Autodesk Fusion 360 part; units mm, degrees
note: some values were not read from the file. Chosen so that the rebuilt part matches the saved one: which bodies a step acts on; which face or edge a step refers to. Set by a fixed rule: which sketch regions a step uses.
(part 2 of 3)
sketch "Sketch13" plane through (0, 0, 15) normal (0, 0, 1) x (-1, 0, 0)
  line L0 (-263, -205.6688) -> (-253, -205.6688)
  line L1 (-253, -205.6688) -> (-253, -217.3312)
  line L2 (-253, -217.3312) -> (-263, -217.3312)
  line L3 (-263, -217.3312) -> (-263, -205.6688)
  line L4 (-263, -137.6688) -> (-253, -137.6688)
  line L5 (-253, -137.6688) -> (-253, -149.3312)
  line L6 (-253, -149.3312) -> (-263, -149.3312)
  line L7 (-263, -149.3312) -> (-263, -137.6688)
  line L8 (-263, -69.6688) -> (-253, -69.6688)
  line L9 (-253, -69.6688) -> (-253, -81.3312)
  line L10 (-253, -81.3312) -> (-263, -81.3312)
  line L11 (-263, -81.3312) -> (-263, -69.6688)
  line L12 (-263, -4) -> (-253, -4)
  line L13 (-253, -4) -> (-253, -13.3312)
  line L14 (-253, -13.3312) -> (-263, -13.3312)
  line L15 (-263, -13.3312) -> (-263, -4)
  line L16 (-263, -52.6688) -> (-253, -52.6688)
  line L17 (-253, -52.6688) -> (-253, -64.3312)
  line L18 (-253, -64.3312) -> (-263, -64.3312)
  line L19 (-263, -64.3312) -> (-263, -52.6688)
  line L20 (-263, -120.6688) -> (-253, -120.6688)
  line L21 (-253, -120.6688) -> (-253, -132.3312)
  line L22 (-253, -132.3312) -> (-263, -132.3312)
  line L23 (-263, -132.3312) -> (-263, -120.6688)
  line L24 (-263, -188.6688) -> (-253, -188.6688)
  line L25 (-253, -188.6688) -> (-253, -200.3312)
  line L26 (-253, -200.3312) -> (-263, -200.3312)
  line L27 (-263, -200.3312) -> (-263, -188.6688)
  line L28 (-263, -222.6688) -> (-253, -222.6688)
  line L29 (-253, -222.6688) -> (-253, -234.3312)
  line L30 (-253, -234.3312) -> (-263, -234.3312)
  line L31 (-263, -234.3312) -> (-263, -222.6688)
  line L32 (-263, -154.6688) -> (-253, -154.6688)
  line L33 (-253, -154.6688) -> (-253, -166.3312)
  line L34 (-253, -166.3312) -> (-263, -166.3312)
  line L35 (-263, -166.3312) -> (-263, -154.6688)
  line L36 (-263, -86.6688) -> (-253, -86.6688)
  line L37 (-253, -86.6688) -> (-253, -98.3312)
  line L38 (-253, -98.3312) -> (-263, -98.3312)
  line L39 (-263, -98.3312) -> (-263, -86.6688)
  line L40 (-263, -18.6688) -> (-253, -18.6688)
  line L41 (-253, -18.6688) -> (-253, -30.3312)
  line L42 (-253, -30.3312) -> (-263, -30.3312)
  line L43 (-263, -30.3312) -> (-263, -18.6688)
  line L44 (-263, -35.6688) -> (-253, -35.6688)
  line L45 (-253, -35.6688) -> (-253, -47.3312)
  line L46 (-253, -47.3312) -> (-263, -47.3312)
  line L47 (-263, -47.3312) -> (-263, -35.6688)
  line L48 (-263, -103.6688) -> (-253, -103.6688)
  line L49 (-253, -103.6688) -> (-253, -115.3312)
  line L50 (-253, -115.3312) -> (-263, -115.3312)
  line L51 (-263, -115.3312) -> (-263, -103.6688)
  line L52 (-263, -171.6688) -> (-253, -171.6688)
  line L53 (-253, -171.6688) -> (-253, -183.3312)
  line L54 (-253, -183.3312) -> (-263, -183.3312)
  line L55 (-263, -183.3312) -> (-263, -171.6688)
  line L56 (-263, -239.6688) -> (-253, -239.6688)
  line L57 (-253, -239.6688) -> (-253, -247)
  line L58 (-253, -247) -> (-263, -247)
  line L59 (-263, -247) -> (-263, -239.6688)
  line L60 (-297, -205.6688) -> (-287, -205.6688)
  line L61 (-287, -205.6688) -> (-287, -217.3312)
  line L62 (-287, -217.3312) -> (-297, -217.3312)
  line L63 (-297, -217.3312) -> (-297, -205.6688)
  line L64 (-297, -137.6688) -> (-287, -137.6688)
  line L65 (-287, -137.6688) -> (-287, -149.3312)
  line L66 (-287, -149.3312) -> (-297, -149.3312)
  line L67 (-297, -149.3312) -> (-297, -137.6688)
  line L68 (-297, -69.6688) -> (-287, -69.6688)
  line L69 (-287, -69.6688) -> (-287, -81.3312)
  line L70 (-287, -81.3312) -> (-297, -81.3312)
  line L71 (-297, -81.3312) -> (-297, -69.6688)
  line L72 (-297, -4) -> (-287, -4)
  line L73 (-287, -4) -> (-287, -13.3312)
  line L74 (-287, -13.3312) -> (-297, -13.3312)
  line L75 (-297, -13.3312) -> (-297, -4)
  line L76 (-297, -52.6688) -> (-287, -52.6688)
  line L77 (-287, -52.6688) -> (-287, -64.3312)
  line L78 (-287, -64.3312) -> (-297, -64.3312)
  line L79 (-297, -64.3312) -> (-297, -52.6688)
  line L80 (-297, -120.6688) -> (-287, -120.6688)
  line L81 (-287, -120.6688) -> (-287, -132.3312)
  line L82 (-287, -132.3312) -> (-297, -132.3312)
  line L83 (-297, -132.3312) -> (-297, -120.6688)
  line L84 (-297, -188.6688) -> (-287, -188.6688)
  line L85 (-287, -188.6688) -> (-287, -200.3312)
  line L86 (-287, -200.3312) -> (-297, -200.3312)
  line L87 (-297, -200.3312) -> (-297, -188.6688)
  line L88 (-297, -222.6688) -> (-287, -222.6688)
  line L89 (-287, -222.6688) -> (-287, -234.3312)
  line L90 (-287, -234.3312) -> (-297, -234.3312)
  line L91 (-297, -234.3312) -> (-297, -222.6688)
  line L92 (-297, -154.6688) -> (-287, -154.6688)
  line L93 (-287, -154.6688) -> (-287, -166.3312)
  line L94 (-287, -166.3312) -> (-297, -166.3312)
  line L95 (-297, -166.3312) -> (-297, -154.6688)
  line L96 (-297, -86.6688) -> (-287, -86.6688)
  line L97 (-287, -86.6688) -> (-287, -98.3312)
  line L98 (-287, -98.3312) -> (-297, -98.3312)
  line L99 (-297, -98.3312) -> (-297, -86.6688)
  line L100 (-297, -18.6688) -> (-287, -18.6688)
  line L101 (-287, -18.6688) -> (-287, -30.3312)
  line L102 (-287, -30.3312) -> (-297, -30.3312)
  line L103 (-297, -30.3312) -> (-297, -18.6688)
  line L104 (-297, -35.6688) -> (-287, -35.6688)
  line L105 (-287, -35.6688) -> (-287, -47.3312)
  line L106 (-287, -47.3312) -> (-297, -47.3312)
  line L107 (-297, -47.3312) -> (-297, -35.6688)
  line L108 (-297, -103.6688) -> (-287, -103.6688)
  line L109 (-287, -103.6688) -> (-287, -115.3312)
  line L110 (-287, -115.3312) -> (-297, -115.3312)
  line L111 (-297, -115.3312) -> (-297, -103.6688)
  line L112 (-297, -171.6688) -> (-287, -171.6688)
  line L113 (-287, -171.6688) -> (-287, -183.3312)
  line L114 (-287, -183.3312) -> (-297, -183.3312)
  line L115 (-297, -183.3312) -> (-297, -171.6688)
  line L116 (-297, -239.6688) -> (-287, -239.6688)
  line L117 (-287, -239.6688) -> (-287, -247)
  line L118 (-287, -247) -> (-297, -247)
  line L119 (-297, -247) -> (-297, -239.6688)
  line L120 (-250, -250) -> (-250, 0)
  line L121 (-250, 0) -> (-300, 0)
  line L122 (-300, 0) -> (-300, -250)
  line L123 (-300, -250) -> (-250, -250)
  line L124 (-257.25, -13.3312) -> (-258.75, -13.3312)
  line L125 (-258.75, -13.3312) -> (-258.75, -154.6688)
  line L126 (-257.25, -13.3312) -> (-257.25, -154.6688)
  line L127 (-258.75, -154.6688) -> (-257.25, -154.6688)
  line L128 (-292.75, -103.6688) -> (-292.75, -239.6688)
  line L129 (-291.25, -103.6688) -> (-291.25, -239.6688)
  line L130 (-292.75, -239.6688) -> (-291.25, -239.6688)
  line L131 (-291.25, -103.6688) -> (-291.25, -98.3312)
  line L132 (-292.75, -103.6688) -> (-292.75, -98.3312)
  line L133 (-292.75, -98.3312) -> (-291.25, -98.3312)
  dimension "d115" = 4.25
  dimension "d120" = 1.5
  dimension "d121" = 1.5
  dimension "d144" = 1.5
  constraint coincident L14 L124.start
  constraint coincident L14 L124.end
  constraint coincident L32 L125.end
  constraint perpendicular L32 L125
  constraint coincident L32 L126.end
  constraint coincident L108 L128.start
  constraint coincident L108 L129.start
  constraint coincident L116 L128.end
  constraint perpendicular L116 L128
  constraint coincident L116 L129.end
  constraint perpendicular L116 L129
  constraint coincident L98 L131.end
  constraint perpendicular L98 L131
  constraint coincident L98 L132.end
  constraint perpendicular L98 L132
  measures "d115" distance of L14.end L124.end
  measures "d120" distance of L125.end L126.end
  measures "d121" distance of L124.start L124.end
  measures "d144" distance of L131.end L132.end
extrude "Extrude15" cut sketch "Sketch13" against normal blind 1 contours L4 L22 L125 L126 | L4 L6 L125 L126 | L20 L22 L125 L126 | L6 L32 L125 L126 L127 | L20 L50 L125 L126 | L48 L50 L125 L126 | L38 L48 L125 L126 | L36 L38 L125 L126 | L10 L36 L125 L126 | L8 L10 L125 L126 | L8 L18 L125 L126 | L16 L18 L125 L126 | L16 L46 L125 L126 | L44 L46 L125 L126 | L42 L44 L125 L126 | L40 L42 L125 L126 | L14 L40 L124 L125 L126 | L60 L86 L128 L129 | L60 L62 L128 L129 | L84 L86 L128 L129 | L62 L88 L128 L129 | L84 L114 L128 L129 | L88 L90 L128 L129 | L112 L114 L128 L129 | L90 L116 L128 L129 L130 | L94 L112 L128 L129 | L92 L94 L128 L129 | L66 L92 L128 L129 | L64 L66 L128 L129 | L64 L82 L128 L129 | L80 L82 L128 L129 | L80 L110 L128 L129 | L108 L110 L128 L129 | L98 L108 L131 L132 L133 bodies 39
sketch "Sketch14" plane through (0, 0, 15) normal (0, 0, 1) x (-1, 0, 0)
  line L0 (-258.75, -154.6688) -> (-258.75, -149.3312)
  line L1 (-258.75, -149.3312) -> (-263, -149.3312)
  line L2 (-263, -149.3312) -> (-263, -137.6688)
  line L3 (-263, -137.6688) -> (-258.75, -137.6688)
  line L4 (-258.75, -137.6688) -> (-258.75, -132.3312)
  line L5 (-258.75, -132.3312) -> (-263, -132.3312)
  line L6 (-263, -132.3312) -> (-263, -120.6688)
  line L7 (-263, -120.6688) -> (-258.75, -120.6688)
  line L8 (-258.75, -120.6688) -> (-258.75, -115.3312)
  line L9 (-258.75, -115.3312) -> (-263, -115.3312)
  line L10 (-263, -115.3312) -> (-263, -103.6688)
  line L11 (-263, -103.6688) -> (-258.75, -103.6688)
  line L12 (-258.75, -103.6688) -> (-258.75, -98.3312)
  line L13 (-258.75, -98.3312) -> (-263, -98.3312)
  line L14 (-263, -98.3312) -> (-263, -86.6688)
  line L15 (-263, -86.6688) -> (-258.75, -86.6688)
  line L16 (-258.75, -86.6688) -> (-258.75, -81.3312)
  line L17 (-258.75, -81.3312) -> (-263, -81.3312)
  line L18 (-263, -81.3312) -> (-263, -69.6688)
  line L19 (-263, -69.6688) -> (-258.75, -69.6688)
  line L20 (-258.75, -69.6688) -> (-258.75, -64.3312)
  line L21 (-258.75, -64.3312) -> (-263, -64.3312)
  line L22 (-263, -64.3312) -> (-263, -52.6688)
  line L23 (-263, -52.6688) -> (-258.75, -52.6688)
  line L24 (-258.75, -52.6688) -> (-258.75, -47.3312)
  line L25 (-258.75, -47.3312) -> (-263, -47.3312)
  line L26 (-263, -47.3312) -> (-263, -35.6688)
  line L27 (-263, -35.6688) -> (-258.75, -35.6688)
  line L28 (-258.75, -35.6688) -> (-258.75, -30.3312)
  line L29 (-258.75, -30.3312) -> (-263, -30.3312)
  line L30 (-263, -30.3312) -> (-263, -18.6688)
  line L31 (-263, -18.6688) -> (-258.75, -18.6688)
  line L32 (-258.75, -18.6688) -> (-258.75, -13.3312)
  line L33 (-258.75, -13.3312) -> (-263, -13.3312)
  line L34 (-263, -13.3312) -> (-263, -4)
  line L35 (-263, -4) -> (-253, -4)
  line L36 (-253, -4) -> (-253, -13.3312)
  line L37 (-253, -13.3312) -> (-257.25, -13.3312)
  line L38 (-257.25, -13.3312) -> (-257.25, -18.6688)
  line L39 (-257.25, -18.6688) -> (-253, -18.6688)
  line L40 (-253, -18.6688) -> (-253, -30.3312)
  line L41 (-253, -30.3312) -> (-257.25, -30.3312)
  line L42 (-257.25, -30.3312) -> (-257.25, -35.6688)
  line L43 (-257.25, -35.6688) -> (-253, -35.6688)
  line L44 (-253, -35.6688) -> (-253, -47.3312)
  line L45 (-253, -47.3312) -> (-257.25, -47.3312)
  line L46 (-257.25, -47.3312) -> (-257.25, -52.6688)
  line L47 (-257.25, -52.6688) -> (-253, -52.6688)
  line L48 (-253, -52.6688) -> (-253, -64.3312)
  line L49 (-253, -64.3312) -> (-257.25, -64.3312)
  line L50 (-257.25, -64.3312) -> (-257.25, -69.6688)
  line L51 (-257.25, -69.6688) -> (-253, -69.6688)
  line L52 (-253, -69.6688) -> (-253, -81.3312)
  line L53 (-253, -81.3312) -> (-257.25, -81.3312)
  line L54 (-257.25, -81.3312) -> (-257.25, -86.6688)
  line L55 (-257.25, -86.6688) -> (-253, -86.6688)
  line L56 (-253, -86.6688) -> (-253, -98.3312)
  line L57 (-253, -98.3312) -> (-257.25, -98.3312)
  line L58 (-257.25, -98.3312) -> (-257.25, -103.6688)
  line L59 (-257.25, -103.6688) -> (-253, -103.6688)
  line L60 (-253, -103.6688) -> (-253, -115.3312)
  line L61 (-253, -115.3312) -> (-257.25, -115.3312)
  line L62 (-257.25, -115.3312) -> (-257.25, -120.6688)
  line L63 (-257.25, -120.6688) -> (-253, -120.6688)
  line L64 (-253, -120.6688) -> (-253, -132.3312)
  line L65 (-253, -132.3312) -> (-257.25, -132.3312)
  line L66 (-257.25, -132.3312) -> (-257.25, -137.6688)
  line L67 (-257.25, -137.6688) -> (-253, -137.6688)
  line L68 (-253, -137.6688) -> (-253, -149.3312)
  line L69 (-253, -149.3312) -> (-257.25, -149.3312)
  line L70 (-257.25, -149.3312) -> (-257.25, -154.6688)
  line L71 (-257.25, -154.6688) -> (-253, -154.6688)
  line L72 (-253, -154.6688) -> (-253, -166.3312)
  line L73 (-253, -166.3312) -> (-263, -166.3312)
  line L74 (-263, -166.3312) -> (-263, -154.6688)
  line L75 (-263, -154.6688) -> (-258.75, -154.6688)
  line L76 (-263, -205.6688) -> (-253, -205.6688)
  line L77 (-253, -205.6688) -> (-253, -217.3312)
  line L78 (-253, -217.3312) -> (-263, -217.3312)
  line L79 (-263, -217.3312) -> (-263, -205.6688)
  line L80 (-263, -188.6688) -> (-253, -188.6688)
  line L81 (-253, -188.6688) -> (-253, -200.3312)
  line L82 (-253, -200.3312) -> (-263, -200.3312)
  line L83 (-263, -200.3312) -> (-263, -188.6688)
  line L84 (-263, -222.6688) -> (-253, -222.6688)
  line L85 (-253, -222.6688) -> (-253, -234.3312)
  line L86 (-253, -234.3312) -> (-263, -234.3312)
  line L87 (-263, -234.3312) -> (-263, -222.6688)
  line L88 (-263, -171.6688) -> (-253, -171.6688)
  line L89 (-253, -171.6688) -> (-253, -183.3312)
  line L90 (-253, -183.3312) -> (-263, -183.3312)
  line L91 (-263, -183.3312) -> (-263, -171.6688)
  line L92 (-263, -239.6688) -> (-253, -239.6688)
  line L93 (-253, -239.6688) -> (-253, -247)
  line L94 (-253, -247) -> (-263, -247)
  line L95 (-263, -247) -> (-263, -239.6688)
  line L96 (-297, -69.6688) -> (-287, -69.6688)
  line L97 (-287, -69.6688) -> (-287, -81.3312)
  line L98 (-287, -81.3312) -> (-297, -81.3312)
  line L99 (-297, -81.3312) -> (-297, -69.6688)
  line L100 (-297, -4) -> (-287, -4)
  line L101 (-287, -4) -> (-287, -13.3312)
  line L102 (-287, -13.3312) -> (-297, -13.3312)
  line L103 (-297, -13.3312) -> (-297, -4)
  line L104 (-297, -52.6688) -> (-287, -52.6688)
  line L105 (-287, -52.6688) -> (-287, -64.3312)
  line L106 (-287, -64.3312) -> (-297, -64.3312)
  line L107 (-297, -64.3312) -> (-297, -52.6688)
  line L108 (-297, -86.6688) -> (-287, -86.6688)
  line L109 (-287, -86.6688) -> (-287, -98.3312)
  line L110 (-292.75, -98.3312) -> (-297, -98.3312)
  line L111 (-297, -98.3312) -> (-297, -86.6688)
  line L112 (-297, -18.6688) -> (-287, -18.6688)
  line L113 (-287, -18.6688) -> (-287, -30.3312)
  line L114 (-287, -30.3312) -> (-297, -30.3312)
  line L115 (-297, -30.3312) -> (-297, -18.6688)
  line L116 (-297, -35.6688) -> (-287, -35.6688)
  line L117 (-287, -35.6688) -> (-287, -47.3312)
  line L118 (-287, -47.3312) -> (-297, -47.3312)
  line L119 (-297, -47.3312) -> (-297, -35.6688)
  line L120 (-292.75, -137.6688) -> (-292.75, -132.3312)
  line L121 (-292.75, -132.3312) -> (-297, -132.3312)
  line L122 (-297, -132.3312) -> (-297, -120.6688)
  line L123 (-297, -120.6688) -> (-292.75, -120.6688)
  line L124 (-292.75, -120.6688) -> (-292.75, -115.3312)
  line L125 (-292.75, -115.3312) -> (-297, -115.3312)
  line L126 (-297, -115.3312) -> (-297, -103.6688)
  line L127 (-297, -103.6688) -> (-292.75, -103.6688)
  line L128 (-287, -103.6688) -> (-287, -115.3312)
  line L129 (-287, -115.3312) -> (-291.25, -115.3312)
  line L130 (-291.25, -98.3312) -> (-291.25, -103.6688)
  line L131 (-291.25, -120.6688) -> (-287, -120.6688)
  line L132 (-287, -120.6688) -> (-287, -132.3312)
  line L133 (-287, -132.3312) -> (-291.25, -132.3312)
  line L134 (-291.25, -132.3312) -> (-291.25, -137.6688)
  line L135 (-291.25, -137.6688) -> (-287, -137.6688)
  line L136 (-287, -137.6688) -> (-287, -149.3312)
  line L137 (-287, -149.3312) -> (-291.25, -149.3312)
  line L138 (-291.25, -149.3312) -> (-291.25, -154.6688)
  line L139 (-291.25, -154.6688) -> (-287, -154.6688)
  line L140 (-287, -154.6688) -> (-287, -166.3312)
  line L141 (-287, -166.3312) -> (-291.25, -166.3312)
  line L142 (-291.25, -166.3312) -> (-291.25, -171.6688)
  line L143 (-291.25, -171.6688) -> (-287, -171.6688)
  line L144 (-287, -171.6688) -> (-287, -183.3312)
  line L145 (-287, -183.3312) -> (-291.25, -183.3312)
  line L146 (-291.25, -183.3312) -> (-291.25, -188.6688)
  line L147 (-291.25, -188.6688) -> (-287, -188.6688)
  line L148 (-287, -188.6688) -> (-287, -200.3312)
  line L149 (-287, -200.3312) -> (-291.25, -200.3312)
  line L150 (-291.25, -200.3312) -> (-291.25, -205.6688)
  line L151 (-291.25, -205.6688) -> (-287, -205.6688)
  line L152 (-287, -205.6688) -> (-287, -217.3312)
  line L153 (-287, -217.3312) -> (-291.25, -217.3312)
  line L154 (-291.25, -217.3312) -> (-291.25, -222.6688)
  line L155 (-291.25, -222.6688) -> (-287, -222.6688)
  line L156 (-287, -222.6688) -> (-287, -234.3312)
  line L157 (-287, -234.3312) -> (-291.25, -234.3312)
  line L158 (-291.25, -234.3312) -> (-291.25, -239.6688)
  line L159 (-291.25, -239.6688) -> (-287, -239.6688)
  line L160 (-287, -239.6688) -> (-287, -247)
  line L161 (-287, -247) -> (-297, -247)
  line L162 (-297, -247) -> (-297, -239.6688)
  line L163 (-297, -239.6688) -> (-292.75, -239.6688)
  line L164 (-292.75, -239.6688) -> (-292.75, -234.3312)
  line L165 (-292.75, -234.3312) -> (-297, -234.3312)
  line L166 (-297, -234.3312) -> (-297, -222.6688)
  line L167 (-297, -222.6688) -> (-292.75, -222.6688)
  line L168 (-292.75, -222.6688) -> (-292.75, -217.3312)
  line L169 (-292.75, -217.3312) -> (-297, -217.3312)
  line L170 (-297, -217.3312) -> (-297, -205.6688)
  line L171 (-297, -205.6688) -> (-292.75, -205.6688)
  line L172 (-292.75, -205.6688) -> (-292.75, -200.3312)
  line L173 (-292.75, -200.3312) -> (-297, -200.3312)
  line L174 (-297, -200.3312) -> (-297, -188.6688)
  line L175 (-297, -188.6688) -> (-292.75, -188.6688)
  line L176 (-292.75, -188.6688) -> (-292.75, -183.3312)
  line L177 (-292.75, -183.3312) -> (-297, -183.3312)
  line L178 (-297, -183.3312) -> (-297, -171.6688)
  line L179 (-297, -171.6688) -> (-292.75, -171.6688)
  line L180 (-292.75, -171.6688) -> (-292.75, -166.3312)
  line L181 (-292.75, -166.3312) -> (-297, -166.3312)
  line L182 (-297, -166.3312) -> (-297, -154.6688)
  line L183 (-297, -154.6688) -> (-292.75, -154.6688)
  line L184 (-292.75, -154.6688) -> (-292.75, -149.3312)
  line L185 (-292.75, -149.3312) -> (-297, -149.3312)
  line L186 (-297, -149.3312) -> (-297, -137.6688)
  line L187 (-297, -137.6688) -> (-292.75, -137.6688)
  line L188 (-250, -250) -> (-250, 0)
  line L189 (-250, 0) -> (-300, 0)
  line L190 (-300, 0) -> (-300, -250)
  line L191 (-300, -250) -> (-250, -250)
  line L192 (-297, -4) -> (-253, -4)
  line L193 (-253, -4) -> (-253, -247)
  line L194 (-253, -247) -> (-297, -247)
  line L195 (-297, -247) -> (-297, -4)
  line L196 (-252, -248) -> (-298, -248)
  line L197 (-298, -248) -> (-298, -3)
  line L198 (-298, -3) -> (-252, -3)
  line L199 (-252, -3) -> (-252, -248)
  line L200 (-287, -4) -> (-287, -247)
  line L201 (-263, -247) -> (-263, -4)
  line L202 (-286, -4) -> (-286, -247)
  line L203 (-264, -247) -> (-264, -4)
  line L204 (-292.75, -103.6688) -> (-292.75, -98.3312)
  line L205 (-287, -98.3312) -> (-291.25, -98.3312)
  line L206 (-291.25, -103.6688) -> (-287, -103.6688)
  line L207 (-291.25, -115.3312) -> (-291.25, -120.6688)
  dimension "d126" = -1
  dimension "d127" = -1
  dimension "d128" = -1
  constraint horizontal L192
  constraint vertical L193
  constraint horizontal L194
  constraint vertical L195
  constraint coincident L93.end L94.start
  constraint coincident L100.start L103.end
  constraint coincident L100.end L101.start
  constraint coincident L160.end L161.start
  constraint coincident L94.end L95.start
  constraint coincident L34.end L35.start
extrude "Extrude16" add sketch "Sketch14" along normal blind 1 contours L2 L6 L10 L14 L18 L22 L26 L30 L34 L74 L79 L83 L87 L91 L95 L192 L194 L201 L203 | L97 L101 L105 L109 L113 L117 L128 L132 L136 L140 L144 L148 L152 L156 L160 L192 L194 L200 L202 | L196 L197 L198 L199 bodies 39
sketch "Sketch15" plane through (0, 0, 15) normal (0, 0, 1) x (-1, 0, 0)
  line L0 (-286, -247) -> (-264, -247)
  line L1 (-264, -247) -> (-264, -4)
  line L2 (-264, -4) -> (-286, -4)
  line L3 (-286, -4) -> (-286, -247)
  line L4 (-287, -234.33) -> (-287, -239.6688)
  line L5 (-287, -239.6688) -> (-291.25, -239.6688)
  line L6 (-291.25, -239.6688) -> (-291.25, -234.33)
  line L7 (-287, -234.33) -> (-291.25, -234.33)
  line L8 (-288, -235.33) -> (-290.25, -235.33)
  line L9 (-290.25, -238.6688) -> (-290.25, -235.33)
  line L10 (-288, -238.6688) -> (-290.25, -238.6688)
  line L11 (-288, -235.33) -> (-288, -238.6688)
  line L12 (-256.25, -153.6688) -> (-256.25, -150.33)
  line L13 (-254, -150.33) -> (-254, -153.6688)
  line L14 (-253, -149.33) -> (-253, -154.6688)
  line L15 (-253, -154.6688) -> (-257.25, -154.6688)
  line L16 (-254, -150.33) -> (-256.25, -150.33)
  line L17 (-253, -149.33) -> (-257.25, -149.33)
  line L18 (-257.25, -154.6688) -> (-257.25, -149.33)
  line L19 (-252, 81) -> (-252, -162)
  line L20 (-254, -153.6688) -> (-256.25, -153.6688)
  dimension "d131" = 5.3388
  dimension "d132" = 4.25
  dimension "d134" = 1
  dimension "d141" = 1
  dimension "d142" = 5.3388
  dimension "d143" = 4.25
  constraint parallel L3 L4
  constraint perpendicular L3 L5
  constraint perpendicular L5 L6
  constraint perpendicular L4 L7
  constraint parallel L14 L19
  constraint perpendicular L15 L19
  constraint perpendicular L15 L18
  constraint perpendicular L14 L17
  measures "d131" distance of L5.end L6.end
  measures "d132" distance of L4.start L6.end
  measures "d142" distance of L15.end L17.end
  measures "d143" distance of L14.start L17.end
extrude "Extrude17" add sketch "Sketch15" along normal blind 1 contours L8 L9 L10 L11 | L12 L13 L16 L20 bodies 39
pattern_linear "R-Pattern2" count 9 spacing 17 along (0, -1, 0) count 2 spacing 5.7 along (1, 0, 0) of "Extrude17"
sketch "Sketch16" plane through (0, 0, 0) normal (0, 0, -1) x (1, 0, 0)
  line L0 (300, -10) -> (300, 0)
  line L1 (300, 0) -> (287, 0)
  line L2 (300, 0) -> (250, 0)
  line L3 (250, 0) -> (250, -250)
  line L4 (250, -250) -> (300, -250)
  line L5 (300, -250) -> (300, 0)
  line L6 (246, 4) -> (246, -254)
  line L7 (246, -254) -> (304, -254)
  line L8 (304, -254) -> (304, 4)
  line L9 (304, 4) -> (246, 4)
  dimension "d145" = 4
  constraint horizontal L2
  constraint vertical L3
  constraint horizontal L4
  constraint vertical L5
  constraint coincident L0.end L1.start
extrude "Extrude18" add sketch "Sketch16" against normal blind 21 separate body contours L0 L1 L2 L3 L4 L5 | L6 L7 L8 L9 makes body 40
combine "Combine1'" operation cut target body 40 tool bodies 39 keep tools result as body 41 in component "Component"
move_body "Move4" bodies 39 to x (1, 0, 0) y (0, 1, 0) z (0, 0, 1) at (-22.6689, -7.9212, -52.6306)
split "Split3" by plane through (275, 125, 7.5) normal (1, 0, 0) bodies 40 makes body 42 at (284.6667, 82, 0)
move_body "Move1" bodies 41 to x (1, 0, 0) y (0, 1, 0) z (0, 0, 1) at (-137.3731, 35.75, -72.9165) in component "Component"
split "Split1" by plane through (112.6269, 35.75, -57.9165) normal (0, 0, -1) bodies 41 makes body 55 at (133.6269, 151.75, -72.9165) makes body 43 at (122.2936, 278.0879, -65.2499) makes body 54 at (118.9603, 267.412, -65.2499) makes body 53 at (118.9603, 244.0879, -65.2499) makes body 51 at (118.9603, 233.412, -65.2499) makes body 49 at (118.9603, 210.0879, -65.2499) makes body 47 at (118.9603, 199.412, -65.2499) makes body 47 at (120.3769, 114.2907, -65.5832) makes body 47 at (120.3769, 46.412, -65.2499) makes body 44 at (156.2936, 46.412, -65.2499) makes body 48 at (156.2936, 57.0879, -65.2499) makes body 46 at (156.2936, 74.0879, -65.2499) makes body 50 at (156.2936, 91.0879, -65.2499) makes body 52 at (156.2936, 114.412, -65.2499) makes body 45 at (156.2936, 125.0879, -65.2499) makes body 45 at (154.3769, 267.2907, -65.5832) makes body 45 at (154.8769, 278.0879, -65.2499) in component "Component"
move_body "Move2" bodies 55 to x (-1, 0, 0) y (0, 1, 0) z (0, 0, -1) at (190.1264, 20.1178, -160.1383) in component "Component"
delete_body "RemoveBody2" bodies 40
delete_body "RemoveBody3" bodies 42
ref_plane "WorkPlane4" through (52.4994, 180.8678, -47.2217) normal (0, 0, 1) x (-1, 0, 0)
combine "Combine2" operation add target body 47 tool bodies 41 45 44 48 43 49 52 46 51 53 50 54 in component "Component"
move_body "Move3" bodies 47 to x (1, 0, 0) y (0, -1, 0) z (0, 0, -1) at (0, 376.5599, -103.8331) in component "Component"
sketch "Sketch20" plane through (0, 0, -47.2217) normal (0, 0, 1) x (1, 0, 0)
  line L0 (77.4994, 55.8678) -> (27.4994, 55.8678)
  line L1 (27.4994, 55.8678) -> (27.4994, 305.8678)
  line L2 (27.4994, 305.8678) -> (77.4994, 305.8678)
  line L3 (77.4994, 305.8678) -> (77.4994, 55.8678)
  dimension "d153" = 50
  dimension "d154" = 250
  constraint horizontal L0
  constraint vertical L1
  constraint horizontal L2
  constraint vertical L3
  measures "d153" distance of L1.end L2.end
  measures "d154" distance of L0.end L1.end
extrude "Extrude20" add sketch "Sketch20" along normal blind 2.5 separate body makes body 56
fillet "Fillet1" radius 15 2 edges at (27.4994, 180.8678, -44.7217) (77.4994, 180.8678, -44.7217) on bodies 56
move_body "Move7" bodies 56 to x (-1, 0, 0) y (0, 1, 0) z (0, 0, -1) at (87.0021, 0, -89.4434)
sketch "Sketch22" plane through (0, 0, -42.2217) normal (0, 0, 1) x (-1, 0, 0)
  line L0 (-59.5027, -305.8678) -> (-9.5027, -305.8678)
  line L1 (-9.5027, -305.8678) -> (-9.5027, -55.8678)
  line L2 (-9.5027, -55.8678) -> (-59.5027, -55.8678)
  line L3 (-59.5027, -55.8678) -> (-59.5027, -305.8678)
  line L4 (-59.5027, -55.8678) -> (-9.5027, -55.8678)
  line L5 (-9.5027, -55.8678) -> (-9.5027, -305.8678)
  line L6 (-9.5027, -305.8678) -> (-59.5027, -305.8678)
  line L7 (-59.5027, -305.8678) -> (-59.5027, -55.8678)
  line L8 (-62.5027, -308.8678) -> (-62.5027, -52.8678)
  line L9 (-62.5027, -52.8678) -> (-6.5027, -52.8678)
  line L10 (-6.5027, -52.8678) -> (-6.5027, -308.8678)
  line L11 (-6.5027, -308.8678) -> (-62.5027, -308.8678)
  dimension "d160" = -3
  constraint horizontal L4
  constraint vertical L5
  constraint horizontal L6
  constraint vertical L7
  constraint coincident L0.end L1.start
  constraint coincident L2.end L3.start
extrude "Extrude22" add sketch "Sketch22" against normal blind 6 separate body contours L0 L1 L2 L3 L4 L5 L6 L7 | L8 L9 L10 L11 makes body 57
combine "Combine4" operation cut target body 57 tool bodies 56 keep tools
move_body "Move8" bodies 56 to x (-1, 0, 0) y (0, 1, 0) z (0, 0, -1) at (258.5331, -85.2699, -67.3692)
sketch "Sketch23" plane through (0, 0, -102.2217) normal (0, 0, -1) x (1, 0, 0)
  line L0 (77.4994, -305.8678) -> (27.4994, -305.8678)
  line L1 (27.4994, -305.8678) -> (27.4994, -55.8678)
  line L2 (27.4994, -55.8678) -> (77.4994, -55.8678)
  line L3 (77.4994, -55.8678) -> (77.4994, -305.8678)
  line L4 (81.4994, -309.8678) -> (81.4994, -51.8678)
  line L5 (81.4994, -51.8678) -> (23.4994, -51.8678)
  line L6 (23.4994, -51.8678) -> (23.4994, -309.8678)
  line L7 (23.4994, -309.8678) -> (81.4994, -309.8678)
  circle A0 centre (78.9994, -54.3678) radius 1
  circle A1 centre (25.9994, -54.3678) radius 1
  circle A2 centre (78.9994, -307.3678) radius 1
  circle A3 centre (25.9994, -307.3678) radius 1
  dimension "d163" = 2.5
  dimension "d164" = 2.5
  dimension "d165" = 2
  dimension "d168" = -53
  dimension "d169" = -253
  measures "d163" distance of L4 A0.centre
  measures "d164" distance of L5 A0.centre
  measures "d165" diameter of A0
extrude "Extrude1'" cut sketch "Sketch23" against normal blind 10 contours A0 | A1 | A2 | A3 bodies 55 in component "Component"
sketch "Sketch24" plane through (0, 0, -45.9166) normal (0, 0, 1) x (-1, 0, 0)
  line L0 (-108.6269, -344.81) -> (-108.6269, -86.81)
  line L1 (-108.6269, -86.81) -> (-166.6269, -86.81)
  line L2 (-166.6269, -86.81) -> (-166.6269, -344.81)
  line L3 (-166.6269, -344.81) -> (-108.6269, -344.81)
  line L4 (-114.6269, -92.81) -> (-114.6269, -337.81)
  line L5 (-114.6269, -337.81) -> (-160.6269, -337.81)
  line L6 (-160.6269, -337.81) -> (-160.6269, -92.81)
  line L7 (-160.6269, -92.81) -> (-114.6269, -92.81)
  circle A0 centre (-164.1269, -89.31) radius 0.925
  circle A1 centre (-111.1269, -89.31) radius 0.925
  circle A2 centre (-164.1269, -342.31) radius 0.925
  circle A3 centre (-111.1269, -342.31) radius 0.925
  dimension "d172" = 1.85
  dimension "d173" = 2.5
  dimension "d174" = 2.5
  dimension "d177" = 53
  dimension "d178" = -253
  measures "d172" diameter of A0
  measures "d173" distance of L1 A0.centre
  measures "d174" distance of L2 A0.centre
extrude "Extrude2'" add sketch "Sketch24" along normal blind 9.5 contours A0 | A1 | A2 | A3 bodies 47 in component "Component"
delete_body "RemoveBody4" bodies 38
delete_body "RemoveBody5" bodies 37
delete_body "RemoveBody6" bodies 36
delete_body "RemoveBody7" bodies 35
delete_body "RemoveBody8" bodies 34
delete_body "RemoveBody9" bodies 33
delete_body "RemoveBody10" bodies 32
delete_body "RemoveBody11" bodies 31
delete_body "RemoveBody12" bodies 30
delete_body "RemoveBody13" bodies 29
delete_body "RemoveBody14" bodies 28
delete_body "RemoveBody15" bodies 27
delete_body "RemoveBody16" bodies 26
delete_body "RemoveBody17" bodies 25
delete_body "RemoveBody18" bodies 24
delete_body "RemoveBody19" bodies 23
delete_body "RemoveBody20" bodies 22
delete_body "RemoveBody21" bodies 21
delete_body "RemoveBody22" bodies 20
delete_body "RemoveBody23" bodies 19
delete_body "RemoveBody24" bodies 18
delete_body "RemoveBody25" bodies 16
delete_body "RemoveBody26" bodies 17
delete_body "RemoveBody27" bodies 1
delete_body "RemoveBody28" bodies 11
delete_body "RemoveBody29" bodies 12
delete_body "RemoveBody30" bodies 13
delete_body "RemoveBody31" bodies 14
delete_body "RemoveBody32" bodies 15
move_body "Move4'" bodies 55 to x (1, 0, 0) y (0, 1, 0) z (0, 0, 1) at (85.0461, 34.5621, 56.9045) in component "Component"
move_body "Move10" bodies 56 to x (1, 0, 0) y (0, 1, 0) z (0, 0, 1) at (28.3007, 21.481, -12.4831)
move_body "Move6" bodies 55 to x (1, 0, 0) y (0, 1, 0) z (0, 0, 1) at (-25.3306, -90.1769, 49.3355) in component "Component"
move_body "Move11" bodies 56 to x (1, 0, 0) y (0, 1, 0) z (0, 0, 1) at (-235.3202, -99.4985, 135.8217)
move_body "Move12" bodies 56 to x (1, 0, 0) y (0, 1, 0) z (0, 0, 1) at (235, 100, -136)
move_body "Move13" bodies 56 to x (1, 0, 0) y (0, 1, 0) z (0, 0, 1) at (-212.7381, 45.3282, 54.3271)
extrude "Extrude23" add 5 faces at (236.9978, 160.1892, -37.6306) (233.6644, 177.1892, -37.6306) (233.6644, 194.1892, -37.6306) (233.6644, 211.1892, -37.6306) (233.6644, 228.1892, -37.6306) along direction (0, 0, 1) up to surface end surface through (-22.6689, -7.9212, -36.6306) normal (0, 0, 1) offset 0 on bodies 39 bodies 39
extrude "Extrude24" add 5 faces at (270.9978, 75.1892, -37.6306) (267.6644, 58.1892, -37.6306) (267.6644, 41.1892, -37.6306) (267.6644, 24.1892, -37.6306) (267.6644, 7.1892, -37.6306) along direction (0, 0, 1) up to surface end surface through (-22.6689, -7.9212, -36.6306) normal (0, 0, 1) offset 0 on bodies 39 bodies 39
extrude "Extrude25" add 1 faces at (248.6644, 77.0788, -37.6306) along direction (0, 0, 1) up to surface (1 mm away) on bodies 39 bodies 39
sketch "Sketch27" plane through (0, 0, -37.6306) normal (0, 0, 1) x (-1, 0, 0)
  line L0 (-227.3311, -242.0788) -> (-227.3311, 7.9212)
  line L1 (-227.3311, 7.9212) -> (-277.3311, 7.9212)
  line L2 (-277.3311, 7.9212) -> (-277.3311, -242.0788)
  line L3 (-277.3311, -242.0788) -> (-227.3311, -242.0788)
  line L4 (-229.3311, 4.9212) -> (-229.3311, -240.0788)
  line L5 (-229.3311, -240.0788) -> (-275.3311, -240.0788)
  line L6 (-275.3311, -240.0788) -> (-275.3311, 4.9212)
  line L7 (-275.3311, 4.9212) -> (-229.3311, 4.9212)
  line L8 (-285.3311, -250.0788) -> (-219.3311, -250.0788)
  line L9 (-219.3311, -250.0788) -> (-219.3311, 15.9212)
  line L10 (-219.3311, 15.9212) -> (-285.3311, 15.9212)
  line L11 (-285.3311, 15.9212) -> (-285.3311, -250.0788)
  dimension "d188" = 8
extrude "Extrude26" add sketch "Sketch27" against normal blind 2 contours L8 L9 L10 L11 bodies 39
sketch "Sketch28" plane through (0, 0, -37.6306) normal (0, 0, 1) x (-1, 0, 0)
  spline S0 degree 5 poles (-281, -14) (-281.6977, -14.6977) (-282.9408, -16.1019) (-284.349, -18.2348) (-285.3213, -21.0853) (-285.1001, -24.4243) (-283.6578, -27.3328) (-281.3643, -29.7132) (-279.0087, -31.8262) (-277.5287, -34.1742) (-277.2439, -36.9195) (-278.0887, -39.5081) (-279.3163, -41.6693) (-280.3953, -43.207) (-281, -44) knots 0 0 0 0 0 0 0.1 0.2 0.3 0.4 0.5 0.6 0.7 0.8 0.9 1 1 1 1 1 1
  spline S1 degree 5 poles (-281, -44) (-281.6977, -44.6977) (-282.9408, -46.1019) (-284.349, -48.2348) (-285.3213, -51.0853) (-285.1001, -54.4243) (-283.6578, -57.3328) (-281.3643, -59.7132) (-279.0087, -61.8262) (-277.5287, -64.1742) (-277.2439, -66.9195) (-278.0887, -69.5081) (-279.3163, -71.6693) (-280.3953, -73.207) (-281, -74) knots 0 0 0 0 0 0 0.1 0.2 0.3 0.4 0.5 0.6 0.7 0.8 0.9 1 1 1 1 1 1
  spline S2 degree 5 poles (-281, -74) (-281.6977, -74.6977) (-282.9408, -76.1019) (-284.349, -78.2348) (-285.3213, -81.0853) (-285.1001, -84.4243) (-283.6578, -87.3328) (-281.3643, -89.7132) (-279.0087, -91.8262) (-277.5287, -94.1742) (-277.2439, -96.9195) (-278.0887, -99.5081) (-279.3163, -101.6693) (-280.3953, -103.207) (-281, -104) knots 0 0 0 0 0 0 0.1 0.2 0.3 0.4 0.5 0.6 0.7 0.8 0.9 1 1 1 1 1 1
  spline S3 degree 5 poles (-281, -104) (-281.6977, -104.6977) (-282.9408, -106.1019) (-284.349, -108.2348) (-285.3213, -111.0853) (-285.1001, -114.4243) (-283.6578, -117.3328) (-281.3643, -119.7132) (-279.0087, -121.8262) (-277.5287, -124.1742) (-277.2439, -126.9195) (-278.0887, -129.5081) (-279.3163, -131.6693) (-280.3953, -133.207) (-281, -134) knots 0 0 0 0 0 0 0.1 0.2 0.3 0.4 0.5 0.6 0.7 0.8 0.9 1 1 1 1 1 1
  spline S4 degree 5 poles (-281, -134) (-281.6977, -134.6977) (-282.9408, -136.1019) (-284.349, -138.2348) (-285.3213, -141.0853) (-285.1001, -144.4243) (-283.6578, -147.3328) (-281.3643, -149.7132) (-279.0087, -151.8262) (-277.5287, -154.1742) (-277.2439, -156.9195) (-278.0887, -159.5081) (-279.3163, -161.6693) (-280.3953, -163.207) (-281, -164) knots 0 0 0 0 0 0 0.1 0.2 0.3 0.4 0.5 0.6 0.7 0.8 0.9 1 1 1 1 1 1
  spline S5 degree 5 poles (-281, -164) (-281.6977, -164.6977) (-282.9408, -166.1019) (-284.349, -168.2348) (-285.3213, -171.0853) (-285.1001, -174.4243) (-283.6578, -177.3328) (-281.3643, -179.7132) (-279.0087, -181.8262) (-277.5287, -184.1742) (-277.2439, -186.9195) (-278.0887, -189.5081) (-279.3163, -191.6693) (-280.3953, -193.207) (-281, -194) knots 0 0 0 0 0 0 0.1 0.2 0.3 0.4 0.5 0.6 0.7 0.8 0.9 1 1 1 1 1 1
  spline S6 degree 5 poles (-281, -194) (-281.6977, -194.6977) (-282.9408, -196.1019) (-284.349, -198.2348) (-285.3213, -201.0853) (-285.1001, -204.4243) (-283.6578, -207.3328) (-281.3643, -209.7132) (-279.0087, -211.8262) (-277.5287, -214.1742) (-277.2439, -216.9195) (-278.0887, -219.5081) (-279.3163, -221.6693) (-280.3953, -223.207) (-281, -224) knots 0 0 0 0 0 0 0.1 0.2 0.3 0.4 0.5 0.6 0.7 0.8 0.9 1 1 1 1 1 1
  spline S7 degree 5 poles (-281, -224) (-281.6977, -224.6977) (-282.9408, -226.1019) (-284.349, -228.2348) (-285.3213, -231.0853) (-285.1001, -234.4243) (-283.6578, -237.3328) (-281.3643, -239.7132) (-279.0087, -241.8262) (-277.5287, -244.1742) (-277.2439, -246.9195) (-278.0887, -249.5081) (-279.3163, -251.6693) (-280.3953, -253.207) (-281, -254) knots 0 0 0 0 0 0 0.1 0.2 0.3 0.4 0.5 0.6 0.7 0.8 0.9 1 1 1 1 1 1
  spline S8 degree 5 poles (-284.423, 11) (-283.9675, 11.6269) (-282.9967, 12.6902) (-281.3618, 13.7141) (-278.9468, 14.0495) (-276.163, 13.3548) (-274.1093, 12.1711) (-273.0331, 11.0447) (-272.0217, 9.9347) (-270.0405, 8.7409) (-267.3285, 8.0162) (-264.9659, 8.3194) (-263.3757, 9.3238) (-262.438, 10.3772) (-262, 11) knots 0 0 0 0 0 0 0.1 0.2 0.3 0.4 0.5 0.6 0.7 0.8 0.9 1 1 1 1 1 1
  line L0 (-274, 11.9999) -> (-272, 10.0001)
  spline S9 degree 5 poles (-284.423, 11) (-284.5806, 10.5896) (-284.9405, 9.4788) (-285.2295, 7.6931) (-284.9797, 5.3329) (-283.6578, 2.6672) (-281.3643, 0.2868) (-279.0087, -1.8262) (-277.5287, -4.1742) (-277.2439, -6.9195) (-278.0887, -9.5081) (-279.3163, -11.6693) (-280.3953, -13.207) (-281, -14) knots 0.141747 0.141747 0.141747 0.141747 0.141747 0.141747 0.2 0.3 0.4 0.5 0.6 0.7 0.8 0.9 1 1 1 1 1 1
  line L1 (-283.2517, 14.0516) -> (-285.5943, 7.9484)
  line L2 (-283.0208, 2.0208) -> (-278.9792, -2.0208)
  line L3 (-252.5, -250) -> (-252.5, -221)
  spline S10 degree 5 poles (-224, -14) (-223.3024, -14.6977) (-222.0592, -16.1019) (-220.651, -18.2348) (-219.6787, -21.0853) (-219.8999, -24.4243) (-221.3422, -27.3328) (-223.6357, -29.7132) (-225.9913, -31.8262) (-227.4713, -34.1742) (-227.7561, -36.9195) (-226.9113, -39.5081) (-225.6837, -41.6693) (-224.6047, -43.207) (-224, -44) knots 0 0 0 0 0 0 0.1 0.2 0.3 0.4 0.5 0.6 0.7 0.8 0.9 1 1 1 1 1 1
  line L4 (-277.7515, -10.7515) -> (-284.2485, -17.2485)
  line L5 (-277.8555, -39.8759) -> (-284.1445, -48.1241)
  line L6 (-227.2485, -10.7515) -> (-220.7515, -17.2485)
  line L7 (-227.1445, -39.8759) -> (-220.8555, -48.1241)
  spline S11 degree 5 poles (-224, -194) (-223.3024, -194.6977) (-222.0592, -196.1019) (-220.651, -198.2348) (-219.6787, -201.0853) (-219.8999, -204.4243) (-221.3422, -207.3328) (-223.6357, -209.7132) (-225.9913, -211.8262) (-227.4713, -214.1742) (-227.7561, -216.9195) (-226.9113, -219.5081) (-225.6837, -221.6693) (-224.6047, -223.207) (-224, -224) knots 0 0 0 0 0 0 0.1 0.2 0.3 0.4 0.5 0.6 0.7 0.8 0.9 1 1 1 1 1 1
  line L8 (-277.7515, -190.7515) -> (-284.2485, -197.2485)
  line L9 (-277.8555, -219.8759) -> (-284.1445, -228.1241)
  line L10 (-227.2485, -190.7515) -> (-220.7515, -197.2485)
  line L11 (-227.1445, -219.8759) -> (-220.8555, -228.1241)
  spline S12 degree 5 poles (-224, -104) (-223.3024, -104.6977) (-222.0592, -106.1019) (-220.651, -108.2348) (-219.6787, -111.0853) (-219.8999, -114.4243) (-221.3422, -117.3328) (-223.6357, -119.7132) (-225.9913, -121.8262) (-227.4713, -124.1742) (-227.7561, -126.9195) (-226.9113, -129.5081) (-225.6837, -131.6693) (-224.6047, -133.207) (-224, -134) knots 0 0 0 0 0 0 0.1 0.2 0.3 0.4 0.5 0.6 0.7 0.8 0.9 1 1 1 1 1 1
  line L12 (-277.7515, -100.7515) -> (-284.2485, -107.2485)
  line L13 (-277.8555, -129.8759) -> (-284.1445, -138.1241)
  line L14 (-227.2485, -100.7515) -> (-220.7515, -107.2485)
  line L15 (-227.1445, -129.8759) -> (-220.8555, -138.1241)
  spline S13 degree 5 poles (-224, -164) (-223.3024, -164.6977) (-222.0592, -166.1019) (-220.651, -168.2348) (-219.6787, -171.0853) (-219.8999, -174.4243) (-221.3422, -177.3328) (-223.6357, -179.7132) (-225.9913, -181.8262) (-227.4713, -184.1742) (-227.7561, -186.9195) (-226.9113, -189.5081) (-225.6837, -191.6693) (-224.6047, -193.207) (-224, -194) knots 0 0 0 0 0 0 0.1 0.2 0.3 0.4 0.5 0.6 0.7 0.8 0.9 1 1 1 1 1 1
  line L16 (-277.7515, -160.7515) -> (-284.2485, -167.2485)
  line L17 (-277.8555, -189.8759) -> (-284.1445, -198.1241)
  line L18 (-227.2485, -160.7515) -> (-220.7515, -167.2485)
  line L19 (-227.1445, -189.8759) -> (-220.8555, -198.1241)
  spline S14 degree 5 poles (-220.577, 11) (-220.4195, 10.5896) (-220.0595, 9.4788) (-219.7705, 7.6931) (-220.0203, 5.3329) (-221.3422, 2.6672) (-223.6357, 0.2868) (-225.9913, -1.8262) (-227.4713, -4.1742) (-227.7561, -6.9195) (-226.9113, -9.5081) (-225.6837, -11.6693) (-224.6047, -13.207) (-224, -14) knots 0.141747 0.141747 0.141747 0.141747 0.141747 0.141747 0.2 0.3 0.4 0.5 0.6 0.7 0.8 0.9 1 1 1 1 1 1
  line L20 (-278.1939, -10.3197) -> (-283.8061, -17.6803)
  line L21 (-221.7483, 14.0516) -> (-219.4057, 7.9484)
  line L22 (-221.9792, 2.0208) -> (-226.0208, -2.0208)
  line L23 (-226.8061, -10.3197) -> (-221.1939, -17.6803)
  spline S15 degree 5 poles (-224, -224) (-223.3024, -224.6977) (-222.0592, -226.1019) (-220.651, -228.2348) (-219.6787, -231.0853) (-219.8999, -234.4243) (-221.3422, -237.3328) (-223.6357, -239.7132) (-225.9913, -241.8262) (-227.4713, -244.1742) (-227.7561, -246.9195) (-226.9113, -249.5081) (-225.6837, -251.6693) (-224.6047, -253.207) (-224, -254) knots 0 0 0 0 0 0 0.1 0.2 0.3 0.4 0.5 0.6 0.7 0.8 0.9 1 1 1 1 1 1
  line L24 (-277.7515, -220.7515) -> (-284.2485, -227.2485)
  line L25 (-277.8555, -249.8759) -> (-284.1445, -258.1241)
  line L26 (-227.2485, -220.7515) -> (-220.7515, -227.2485)
  line L27 (-227.1445, -249.8759) -> (-220.8555, -258.1241)
  spline S16 degree 5 poles (-224, -44) (-223.3024, -44.6977) (-222.0592, -46.1019) (-220.651, -48.2348) (-219.6787, -51.0853) (-219.8999, -54.4243) (-221.3422, -57.3328) (-223.6357, -59.7132) (-225.9913, -61.8262) (-227.4713, -64.1742) (-227.7561, -66.9195) (-226.9113, -69.5081) (-225.6837, -71.6693) (-224.6047, -73.207) (-224, -74) knots 0 0 0 0 0 0 0.1 0.2 0.3 0.4 0.5 0.6 0.7 0.8 0.9 1 1 1 1 1 1
  line L28 (-277.7515, -40.7515) -> (-284.2485, -47.2485)
  line L29 (-277.8555, -69.8759) -> (-284.1445, -78.1241)
  line L30 (-227.2485, -40.7515) -> (-220.7515, -47.2485)
  line L31 (-227.1445, -69.8759) -> (-220.8555, -78.1241)
  spline S17 degree 5 poles (-224, -134) (-223.3024, -134.6977) (-222.0592, -136.1019) (-220.651, -138.2348) (-219.6787, -141.0853) (-219.8999, -144.4243) (-221.3422, -147.3328) (-223.6357, -149.7132) (-225.9913, -151.8262) (-227.4713, -154.1742) (-227.7561, -156.9195) (-226.9113, -159.5081) (-225.6837, -161.6693) (-224.6047, -163.207) (-224, -164) knots 0 0 0 0 0 0 0.1 0.2 0.3 0.4 0.5 0.6 0.7 0.8 0.9 1 1 1 1 1 1
  line L32 (-277.7515, -130.7515) -> (-284.2485, -137.2485)
  line L33 (-277.8555, -159.8759) -> (-284.1445, -168.1241)
  line L34 (-227.2485, -130.7515) -> (-220.7515, -137.2485)
  line L35 (-227.1445, -159.8759) -> (-220.8555, -168.1241)
  spline S18 degree 5 poles (-224, -74) (-223.3024, -74.6977) (-222.0592, -76.1019) (-220.651, -78.2348) (-219.6787, -81.0853) (-219.8999, -84.4243) (-221.3422, -87.3328) (-223.6357, -89.7132) (-225.9913, -91.8262) (-227.4713, -94.1742) (-227.7561, -96.9195) (-226.9113, -99.5081) (-225.6837, -101.6693) (-224.6047, -103.207) (-224, -104) knots 0 0 0 0 0 0 0.1 0.2 0.3 0.4 0.5 0.6 0.7 0.8 0.9 1 1 1 1 1 1
  line L36 (-277.7515, -70.7515) -> (-284.2485, -77.2485)
  line L37 (-277.8555, -99.8759) -> (-284.1445, -108.1241)
  line L38 (-227.2485, -70.7515) -> (-220.7515, -77.2485)
  line L39 (-227.1445, -99.8759) -> (-220.8555, -108.1241)
  spline S19 degree 5 poles (-220.577, 11) (-221.0325, 11.6269) (-222.0033, 12.6902) (-223.6382, 13.7141) (-226.0532, 14.0495) (-228.837, 13.3548) (-230.8907, 12.1711) (-231.9669, 11.0447) (-232.9783, 9.9347) (-234.9596, 8.7409) (-237.6716, 8.0162) (-240.0341, 8.3194) (-241.6243, 9.3238) (-242.562, 10.3772) (-243, 11) knots 0 0 0 0 0 0 0.1 0.2 0.3 0.4 0.5 0.6 0.7 0.8 0.9 1 1 1 1 1 1
  line L40 (-286.3297, 8.3759) -> (-282.5163, 13.6241)
  line L41 (-263.862, 8.3527) -> (-260.138, 13.6473)
  line L42 (-218.6703, 8.3759) -> (-222.4837, 13.6241)
  line L43 (-231, 11.9999) -> (-233, 10.0001)
  line L44 (-241.138, 8.3527) -> (-244.862, 13.6473)
  spline S20 degree 5 poles (-262, 11) (-261.6445, 11.3757) (-260.9314, 12.094) (-259.8553, 13.0722) (-258.4073, 14.1745) (-256.5738, 15.1934) (-254.7148, 15.8222) (-252.8284, 16.0305) (-250.9137, 15.8048) (-248.9719, 15.1654) (-247.0053, 14.145) (-245.4138, 13.0495) (-244.2106, 12.081) (-243.4042, 11.371) (-243, 11) knots 0 0 0 0 0 0 0.1 0.2 0.3 0.4 0.5 0.6 0.7 0.8 0.9 1 1 1 1 1 1
  line L45 (-219.3311, 15.9212) -> (-285.3311, 15.9212)
  line L46 (-281, -254) -> (-224, -254)
  line L47 (-295, 25) -> (-210, 25)
  line L48 (-210, 25) -> (-210, -260)
  line L49 (-210, -260) -> (-295, -260)
  line L50 (-295, -260) -> (-295, 25)
  point P0 (-281, 0)
  point P1 (-279, -32)
  point P2 (-281, -30)
  point P3 (-279, -62)
  point P4 (-281, -60)
  point P5 (-279, -92)
  point P6 (-281, -90)
  point P7 (-279, -122)
  point P8 (-281, -120)
  point P9 (-279, -152)
  point P10 (-281, -150)
  point P11 (-279, -182)
  point P12 (-281, -180)
  point P13 (-279, -212)
  point P14 (-281, -210)
  point P15 (-279, -242)
  point P16 (-281, -240)
  point P17 (-273, 11)
  point P18 (-226, -182)
  point P19 (-220, -250)
  point P20 (-232, 11)
  point P21 (-224, -180)
  point P22 (-226, -32)
  point P23 (-226, -122)
  point P24 (-224, -150)
  point P25 (-224, -90)
  point P26 (-224, 0)
  point P27 (-224, -120)
  point P28 (-224, -60)
  point P29 (-226, -152)
  point P30 (-226, -92)
  point P31 (-226, -242)
  point P32 (-226, -212)
  point P33 (-224, -210)
  point P34 (-224, 16)
  point P35 (-226, -62)
  point P36 (-224, -240)
  point P37 (-224, -30)
  point P38 (-253, 15.9212)
  dimension "d202" = 57
  constraint midpoint P17 L0
  constraint midpoint S8.start L1
  constraint midpoint P0 L2
  constraint midpoint S0.start L4
  constraint midpoint S0.end L5
  constraint midpoint S5.end L8
  constraint midpoint S6.end L9
  constraint midpoint S2.end L12
  constraint midpoint S3.end L13
  constraint midpoint S4.end L16
  constraint midpoint S5.end L17
  constraint midpoint S0.start L20
  constraint midpoint S6.end L24
  constraint midpoint S7.end L25
  constraint midpoint S0.end L28
  constraint midpoint S1.end L29
  constraint midpoint S3.end L32
  constraint midpoint S4.end L33
  constraint midpoint S1.end L36
  constraint midpoint S2.end L37
  constraint midpoint S8.start L40
  constraint midpoint S8.end L41
  constraint symmetric S0.start L3 S10.start
  constraint symmetric P0 L3 P26
  constraint symmetric P1 L3 P22
  constraint symmetric P2 L3 P37
  constraint symmetric S0.end L3 S10.end
  constraint symmetric P3 L3 P35
  constraint symmetric P4 L3 P28
  constraint symmetric S1.end L3 S16.end
  constraint symmetric P5 L3 P30
  constraint symmetric P6 L3 P25
  constraint symmetric S2.end L3 S12.start
  constraint symmetric P7 L3 P23
  constraint symmetric P8 L3 P27
  constraint symmetric S3.end L3 S12.end
  constraint symmetric P9 L3 P29
  constraint symmetric P10 L3 P24
  constraint symmetric S4.end L3 S13.start
  constraint symmetric P11 L3 P18
  constraint symmetric P12 L3 P21
  constraint symmetric S5.end L3 S11.start
  constraint symmetric P13 L3 P32
  constraint symmetric P14 L3 P33
  constraint symmetric S6.end L3 S11.end
  constraint symmetric P15 L3 P31
  constraint symmetric P16 L3 P36
  constraint symmetric S7.end L3 S15.end
  constraint symmetric S8.start L3 S14.start
  constraint symmetric S8.end L3 S19.end
  constraint symmetric P17 L3 P20
  constraint symmetric L0.start L3 L43.start
  constraint symmetric L0.end L3 L43.end
  constraint symmetric L1.start L3 L21.start
  constraint symmetric L1.end L3 L21.end
  constraint symmetric L2.start L3 L22.start
  constraint symmetric L2.end L3 L22.end
  constraint symmetric L3 L4.start L6.start
  constraint symmetric L3 L4.end L6.end
  constraint symmetric L3 L5.start L7.start
  constraint symmetric L3 L5.end L7.end
  constraint symmetric L3 L8.start L10.start
  constraint symmetric L3 L8.end L10.end
  constraint symmetric L3 L9.start L11.start
  constraint symmetric L3 L9.end L11.end
  constraint symmetric L3 L12.start L14.start
  constraint symmetric L3 L12.end L14.end
  constraint symmetric L3 L13.start L15.start
  constraint symmetric L3 L13.end L15.end
  constraint symmetric L3 L16.start L18.start
  constraint symmetric L3 L16.end L18.end
  constraint symmetric L3 L17.start L19.start
  constraint symmetric L3 L17.end L19.end
  constraint symmetric L3 L20.start L23.start
  constraint symmetric L3 L20.end L23.end
  constraint symmetric L3 L24.start L26.start
  constraint symmetric L3 L24.end L26.end
  constraint symmetric L3 L25.start L27.start
  constraint symmetric L3 L25.end L27.end
  constraint symmetric L3 L28.start L30.start
  constraint symmetric L3 L28.end L30.end
  constraint symmetric L3 L29.start L31.start
  constraint symmetric L3 L29.end L31.end
  constraint symmetric L3 L32.start L34.start
  constraint symmetric L3 L32.end L34.end
  constraint symmetric L3 L33.start L35.start
  constraint symmetric L3 L33.end L35.end
  constraint symmetric L3 L36.start L38.start
  constraint symmetric L3 L36.end L38.end
  constraint symmetric L3 L37.start L39.start
  constraint symmetric L3 L37.end L39.end
  constraint symmetric L3 L40.start L42.start
  constraint symmetric L3 L40.end L42.end
  constraint symmetric L3 L41.start L44.start
  constraint symmetric L3 L41.end L44.end
  constraint horizontal L47
  constraint vertical L48
  constraint horizontal L49
  constraint vertical L50
  measures "d202" distance of S7.end S15.end
ref_plane "WorkPlane5" through (252.3311, 117.0788, -7.6306) normal (0, 0, 1) x (0, -1, 0)
sketch "Sketch29" plane through (0, 0, -7.6306) normal (0, 0, 1) x (1, 0, 0)
  line L0 (285.3742, -15.9257) -> (219.3742, -15.9257)
  line L1 (219.3742, -15.9257) -> (219.3742, 250.0743)
  line L2 (219.3742, 250.0743) -> (285.3742, 250.0743)
  line L3 (285.3742, 250.0743) -> (285.3742, -15.9257)
  dimension "d204" = 66
  dimension "d205" = 266
  constraint horizontal L0
  constraint vertical L1
  constraint horizontal L2
  constraint vertical L3
  measures "d204" distance of L1.end L2.end
  measures "d205" distance of L0.end L1.end
move_face "OffsetFaces2" offset 1 2 faces at (264.6644, -7.9212, -43.9639) (239.9978, -7.9212, -43.9639) on bodies 39
fillet "Fillet2" radius 7 1 edges at (270.8311, -8.9212, -52.6306) on bodies 39
fillet "Fillet2" radius 7 1 edges at (233.8311, -8.9212, -52.6306) on bodies 39
extrude "Extrude29" add 2 faces at (239.9978, 242.0788, -43.9639) (264.6644, 242.0788, -43.9639) along direction (0, 1, 0) blind 4 on bodies 39 bodies 39
fillet "Fillet3" radius 6 1 edges at (270.8311, 246.0788, -52.6306) on bodies 39
fillet "Fillet3" radius 6 1 edges at (233.8311, 246.0788, -52.6306) on bodies 39